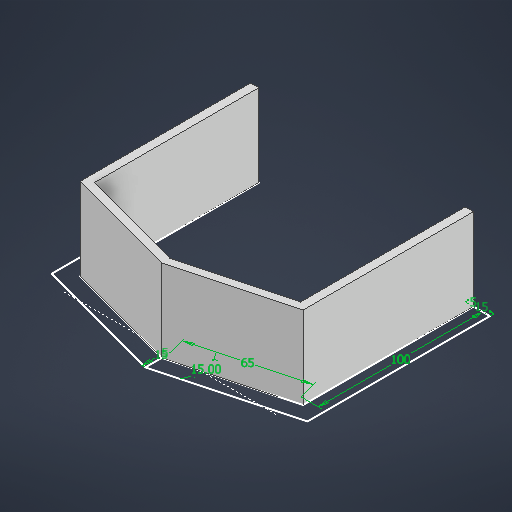
# Autodesk Inventor part: Rumpf
Saved by Autodesk Inventor 2026.2 (Build 302298000, 298)
## iProperties
Created: 2026-01-19
Part Number: Rumpf
Material: Generic
Document SubType Name: Modeling
Designer: Cobble
Density: 1 g/cm^3
Appearance: Default
Author: Cobble
Autodesk Inventor part; units mm, degrees
ref_plane "YZ Plane" through (0, 0, 0) normal (1, 0, 0) x (0, 1, 0)
ref_plane "XZ Plane" through (0, 0, 0) normal (0, 1, 0) x (-1, 0, 0)
ref_plane "XY Plane" through (0, 0, 0) normal (0, 0, 1) x (1, 0, 0)
sketch "Sketch1" plane through (0, 0, 0) normal (0, 0, 1) x (1, 0, 0)
  line L0 (0, 0) -> (62.7852, 16.8232)
  line L1 (0, 0) -> (65, 0) construction
  line L2 (62.7852, 16.8232) -> (62.7852, 116.8232)
  line L3 (62.7852, 116.8232) -> (67.7852, 116.8232)
  line L4 (67.7852, 116.8232) -> (67.7852, 13.163)
  line L5 (67.7852, 13.163) -> (0, -5)
  line L6 (0, -5) -> (0, 0)
  line L7 (0, 0) -> (-62.7852, 16.8232)
  line L8 (0, 0) -> (-65, 0) construction
  line L9 (-62.7852, 16.8232) -> (-62.7852, 116.8232)
  line L10 (-62.7852, 116.8232) -> (-67.7852, 116.8232)
  line L11 (-67.7852, 116.8232) -> (-67.7852, 13.163)
  line L12 (-67.7852, 13.163) -> (0, -5)
  line L13 (0, 0) -> (62.7852, 16.8232)
  line L14 (0, 0) -> (65, 0) construction
  line L15 (62.7852, 16.8232) -> (62.7852, 116.8232)
  line L16 (62.7852, 116.8232) -> (77.7852, 116.8232)
  line L17 (77.7852, 116.8232) -> (77.7852, 5.8425)
  line L18 (77.7852, 5.8425) -> (0, -15)
  line L19 (0, 0) -> (0, -15)
  line L20 (0, 0) -> (-62.7852, 16.8232)
  line L21 (0, 0) -> (-65, 0) construction
  line L22 (-62.7852, 16.8232) -> (-62.7852, 116.8232)
  line L23 (-62.7852, 116.8232) -> (-77.7852, 116.8232)
  line L24 (-77.7852, 116.8232) -> (-77.7852, 5.8425)
  line L25 (-77.7852, 5.8425) -> (0, -15)
  dimension "d0" = 65
  dimension "d1" = 15
  dimension "d2" = 100
  dimension "d3" = 5
  dimension "d4" = 5
  dimension "d7" = 65
  dimension "d8" = 15
  dimension "d9" = 100
  dimension "d10" = 15
  dimension "d11" = 15
  constraints: 52 end point, 10 symmetric about line, 4 perpendicular, 3 parallel, 3 vertical, 2 equal length, 2 horizontal
  measures "d0" distance of L0.start L0.end
  measures "d1" angle of L1 L0
  measures "d2" distance of L0.end L2.end
  measures "d3" distance of L2.end L3.end
  measures "d4" distance of L5.end L0.start
  measures "d7" distance of L13.start L13.end
  measures "d8" angle of L14 L13
  measures "d9" distance of L13.end L15.end
  measures "d10" distance of L15.end L16.end
  measures "d11" distance of L18.end L13.start
extrude "Extrusion1" add sketch "Sketch1" along normal blind 50 contours L0 L2 L3 L4 L5 L6 | L6 L12 L11 L10 L9 L7
body "Solid1"
